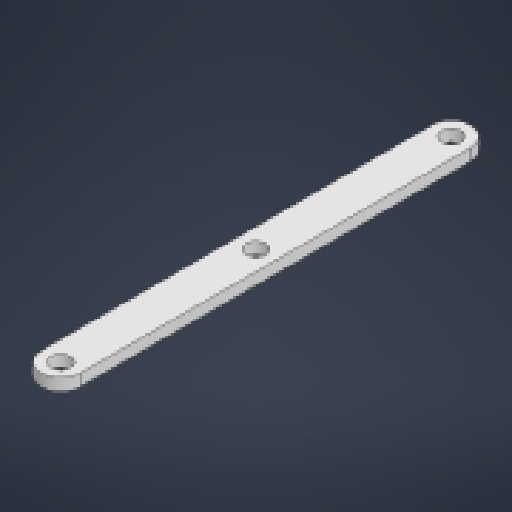
# Autodesk Inventor part: Lazy Tongs beam Long
Saved by Autodesk Inventor 2023.6 (Build 276521000, 521)
## iProperties
Created: 2026-03-05
Part Number: Lazy Tongs beam Long
Material: Generic
Document SubType Name: Modeling
Designer: user
Density: 1 g/cm^3
Appearance: Default
Author: user
Autodesk Inventor part; units mm, degrees
ref_plane "YZ Plane" through (0, 0, 0) normal (1, 0, 0) x (0, 1, 0)
ref_plane "XZ Plane" through (0, 0, 0) normal (0, 1, 0) x (-1, 0, 0)
ref_plane "XY Plane" through (0, 0, 0) normal (0, 0, 1) x (1, 0, 0)
sketch "Sketch1" plane through (0, 0, 0) normal (0, 1, 0) x (-1, 0, 0)
  line L0 (0, 50) -> (0, -50) construction
  line L1 (-5, 50) -> (-5, -50)
  line L2 (5, -50) -> (5, 50)
  arc A0 (5, 50) -> (-5, 50) centre (0, 50) ccw
  arc A1 (-5, -50) -> (5, -50) centre (0, -50) ccw
  circle A2 centre (0, 50) radius 2.5
  circle A3 centre (0, 0) radius 2.5
  circle A4 centre (0, -50) radius 2.5
  dimension "d0" = 50
  dimension "d1" = 10
  dimension "d2" = 5
  dimension "d3" = 5
  dimension "d4" = 5
  constraints: 8 end point, 5 centre point, 4 point on circle, 4 tangent, 3 coincident, 1 midpoint, 1 parallel, 1 vertical
  measures "d0" distance of point (0, 0) L0.end
  measures "d1" diameter of A1
  measures "d2" diameter of A2
  measures "d3" diameter of A3
  measures "d4" diameter of A4
extrude "Extrusion1" add sketch "Sketch1" along normal blind 3
body "Solid1"
